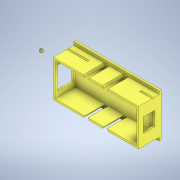
# Autodesk Inventor part: usbHubCaseForTripodClamp
Saved by Autodesk Inventor 2021.2 (Build 252289000, 289)
## iProperties
Created: 2021-02-17
Part Number: usbHubCaseForTripodClamp
Material: PC/ABS Plastic
Document SubType Name: Modeling
Designer: robst
Density: 0.357273 g/cm^3
Appearance: Smooth - Yellow
Author: robst
Autodesk Inventor part; units mm, degrees
ref_plane "YZ Plane" through (0, 0, 0) normal (1, 0, 0) x (0, 1, 0)
ref_plane "XZ Plane" through (0, 0, 0) normal (0, 1, 0) x (-1, 0, 0)
ref_plane "XY Plane" through (0, 0, 0) normal (0, 0, 1) x (1, 0, 0)
sketch "Sketch1" plane through (0, 0, 0) normal (0, 0, 1) x (1, 0, 0)
  line L0 (-57.15, -29.21) -> (57.15, -29.21)
  line L1 (57.15, -29.21) -> (57.15, 29.21)
  line L2 (57.15, 29.21) -> (-57.15, 29.21)
  line L3 (-57.15, 29.21) -> (-57.15, -29.21)
  line L4 (-57.15, -29.21) -> (57.15, 29.21) construction
  line L5 (57.15, -29.21) -> (-57.15, 29.21) construction
  point P0 (0, 0)
  dimension "d0" = 58.42
  dimension "d1" = 114.3
  constraints: 12 end point, 2 midpoint, 2 parallel, 1 horizontal, 1 perpendicular
  measures "d0" distance of L2.end L0.start
  measures "d1" distance of L1.end L2.end
extrude "Extrusion1" add sketch "Sketch1" against normal blind 2.54
sketch "Sketch2" plane through (0, 0, 0) normal (0, 0, 1) x (1, 0, 0)
  line L0 (-57.15, -29.21) -> (-57.15, 29.21) projected
  line L1 (57.15, 29.21) -> (57.15, -29.21) projected
  line L2 (-57.15, 24.765) -> (57.15, 24.765)
  line L3 (57.15, 24.765) -> (57.15, 22.225)
  line L4 (57.15, 22.225) -> (-57.15, 22.225)
  line L5 (-57.15, 22.225) -> (-57.15, 24.765)
  line L6 (-57.15, -24.765) -> (57.15, -24.765)
  line L7 (57.15, -24.765) -> (57.15, -22.225)
  line L8 (57.15, -22.225) -> (-57.15, -22.225)
  line L9 (-57.15, -22.225) -> (-57.15, -24.765)
  point P0 (0, 0)
  point P1 (-57.15, -22.225)
  point P2 (57.15, -24.765)
  dimension "d4" = 2.54
  dimension "d5" = 2.54
  dimension "d6" = 22.225
  dimension "d7" = 22.225
  constraints: 16 end point, 4 parallel, 4 point on line, 2 horizontal, 2 perpendicular
  measures "d4" distance between parallel lines of L4 L2
  measures "d5" distance between parallel lines of L6 L8
  measures "d6" distance from line of L4 point (0, 0)
  measures "d7" distance from line of L8 point (0, 0)
extrude "Extrusion2" add sketch "Sketch2" along normal blind 27.432 contours L0 L8 L1 L6 | L0 L2 L1 L4
sketch "Sketch3" plane through (0, 0, -2.54) normal (0, 0, -1) x (-1, 0, 0)
  line L0 (-12.7, -25.4) -> (12.7, -25.4) construction
  line L1 (12.7, -25.4) -> (12.7, 25.4) construction
  line L2 (12.7, 25.4) -> (-12.7, 25.4) construction
  line L3 (-12.7, 25.4) -> (-12.7, -25.4) construction
  line L4 (-12.7, -25.4) -> (12.7, 25.4) construction
  line L5 (12.7, -25.4) -> (-12.7, 25.4) construction
  point P0 (0, 0)
  dimension "d10" = 25.4
  dimension "d11" = 50.8
  constraints: 12 end point, 4 coincident, 2 midpoint, 2 parallel, 1 horizontal, 1 perpendicular
  measures "d10" distance of L1.end L2.end
  measures "d11" distance of L2.end L0.start
hole "Hole1" at (12.7, 25.4, -2.54) at (-12.7, 25.4, -2.54) at (-12.7, -25.4, -2.54) at (12.7, -25.4, -2.54) direction (0, 0, 1) diameter 3.81 end through all clearance for "Flat Head Machine Screw (82)" size "#6" standard "Ansi Unified Screw Threads"
sketch "Sketch4" plane through (0, 0, 0) normal (0, 0, 1) x (1, 0, 0)
  circle A0 centre (-12.7, 25.4) radius 1.905 projected
  circle A1 centre (-12.7, 25.4) radius 3.81
  circle A2 centre (12.7, 25.4) radius 1.905 projected
  circle A3 centre (12.7, 25.4) radius 3.81
  circle A4 centre (12.7, -25.4) radius 1.905 projected
  circle A5 centre (12.7, -25.4) radius 3.81
  arc A6 (-14.4961, -24.765) -> (-10.9039, -24.765) centre (-12.7, -25.4) ccw projected
  circle A7 centre (-12.7, -25.4) radius 3.81
  point P0 (0, 0)
  dimension "d19" = 7.62
  constraints: 4 centre point, 4 coincident, 3 equal radius
  measures "d19" diameter of A1
extrude "Extrusion3" cut sketch "Sketch4" along normal through all contours A0 | A1 | A2 | A3 | A4 | A5 | A7
sketch "Sketch5" plane through (57.15, -29.21, -2.54) normal (1, 0, 0) x (0, 0, -1)
  line L0 (-29.972, 53.975) -> (-29.972, 51.435) projected
  line L1 (-2.54, 51.435) -> (-2.54, 6.985) projected
  line L2 (-29.972, 51.435) -> (-2.54, 51.435)
  line L3 (-2.54, 51.435) -> (-2.54, 6.985)
  line L4 (-2.54, 6.985) -> (-29.972, 6.985)
  line L5 (-29.972, 6.985) -> (-29.972, 51.435)
  point P0 (-2.54, 29.21)
  constraints: 8 end point, 2 parallel, 1 horizontal, 1 perpendicular
extrude "Extrusion4" add sketch "Sketch5" against normal blind 2.54
sketch "Sketch6" plane through (57.15, -29.21, -2.54) normal (1, 0, 0) x (0, 0, -1)
  line L0 (-2.54, 51.435) -> (-29.972, 51.435) projected
  line L1 (-2.54, 6.985) -> (-2.54, 51.435) projected
  line L2 (-29.972, 6.985) -> (-2.54, 6.985) projected
  line L3 (-29.972, 51.435) -> (-29.972, 53.975) construction
  line L4 (-29.972, 51.435) -> (-2.54, 6.985) construction
  line L5 (-2.54, 51.435) -> (-29.972, 6.985) construction
  line L6 (-23.876, 19.685) -> (-8.636, 19.685)
  line L7 (-8.636, 19.685) -> (-8.636, 38.735)
  line L8 (-8.636, 38.735) -> (-23.876, 38.735)
  line L9 (-23.876, 38.735) -> (-23.876, 19.685)
  line L10 (-23.876, 19.685) -> (-8.636, 38.735) construction
  line L11 (-8.636, 19.685) -> (-23.876, 38.735) construction
  point P0 (-2.54, 29.21)
  point P1 (-16.256, 29.21)
  dimension "d24" = 15.24
  dimension "d25" = 19.05
  constraints: 16 end point, 3 midpoint, 2 parallel, 1 horizontal, 1 perpendicular
  measures "d24" distance of L7.end L8.end
  measures "d25" distance of L6.end L7.end
extrude "Extrusion5" cut sketch "Sketch6" against normal up to surface (2.54 mm away)
sketch "Sketch7" plane through (-57.15, -29.21, -2.54) normal (-1, 0, 0) x (0, 0, 1)
  line L0 (2.54, 51.435) -> (29.972, 51.435) projected
  line L1 (29.972, 6.985) -> (29.972, 51.435) projected
  line L2 (2.54, 6.985) -> (29.972, 6.985) projected
  line L3 (2.54, 51.435) -> (2.54, 6.985) projected
  line L4 (2.54, 6.985) -> (2.54, 51.435) construction
  line L5 (29.972, 6.985) -> (2.54, 6.985) construction
  line L6 (2.54, 51.435) -> (29.972, 6.985) construction
  line L7 (2.54, 51.435) -> (29.972, 51.435) construction
  line L8 (29.972, 51.435) -> (2.54, 6.985) construction
  line L9 (5.461, 13.97) -> (27.051, 13.97)
  line L10 (27.051, 13.97) -> (27.051, 44.45)
  line L11 (27.051, 44.45) -> (5.461, 44.45)
  line L12 (5.461, 44.45) -> (5.461, 13.97)
  line L13 (5.461, 13.97) -> (27.051, 44.45) construction
  line L14 (27.051, 13.97) -> (5.461, 44.45) construction
  point P0 (2.54, 29.21)
  point P1 (16.256, 29.21)
  dimension "d28" = 30.48
  dimension "d29" = 21.59
  constraints: 16 end point, 3 midpoint, 2 parallel, 2 perpendicular
  measures "d28" distance of L11.end L9.start
  measures "d29" distance of L10.end L11.end
extrude "Extrusion6" add sketch "Sketch7" against normal blind 2.54
sketch "Sketch8" plane through (57.15, -29.21, -2.54) normal (1, 0, 0) x (0, 0, -1)
  line L0 (-2.54, 53.975) -> (-29.972, 53.975) projected
  line L1 (-29.972, 53.975) -> (-2.54, 53.975) projected
  line L2 (-12.192, 53.975) -> (-10.922, 52.705)
  line L3 (-10.922, 52.705) -> (-9.652, 53.975)
  line L4 (-9.652, 53.975) -> (-12.192, 53.975)
  line L5 (-29.972, 4.445) -> (-29.972, 53.975) projected
  point P0 (-2.54, 29.21)
  dimension "d32" = 90
  dimension "d33" = 135
  dimension "d34" = 1.27
  dimension "d35" = 19.05
  constraints: 6 end point, 2 point on line, 1 collinear
  measures "d32" angle of L3 L2
  measures "d33" angle of L2 L0
  measures "d34" distance from line of L2.end L0
  measures "d35" distance from line of L2.end L5
extrude "Extrusion7" cut sketch "Sketch8" against normal blind 16.51
mirror "Mirror1" about plane through (0, 0, 0) normal (0, 1, 0) of "Extrusion7"
sketch "Sketch9" plane through (-57.15, -29.21, -2.54) normal (-1, 0, 0) x (0, 0, 1)
  line L0 (9.652, 53.975) -> (10.922, 52.705) projected
  line L1 (10.922, 52.705) -> (12.192, 53.975) projected
  line L2 (2.54, 53.975) -> (29.972, 53.975) projected
  line L3 (12.192, 53.975) -> (10.922, 52.705)
  line L4 (9.652, 53.975) -> (10.922, 52.705) projected
  line L5 (10.922, 52.705) -> (9.652, 53.975)
  line L6 (9.652, 53.975) -> (12.192, 53.975)
  line L7 (2.54, 53.975) -> (29.972, 53.975) projected
  point P0 (2.54, 29.21)
  constraints: 6 end point, 2 collinear
extrude "Extrusion8" cut sketch "Sketch9" against normal blind 27.94
mirror "Mirror2" about plane through (0, 0, 0) normal (0, 1, 0) of "Extrusion8"
equation "\"d0\" = usbHolderWidth"
equation "\"d1\" = usbHolderLength"
equation "\"d2\" = usbHolderWallThickness"
equation "\"d4\" = usbHolderWallThickness"
equation "\"d5\" = usbHolderWallThickness"
equation "\"d6\" = 0.5 * usbHubWidth"
equation "\"d7\" = 0.5 * usbHubWidth"
equation "\"d8\" = usbHubDepth"
equation "\"d10\" = holePatternLength"
equation "\"d11\" = holePatternWidth"
equation "\"d22\" = usbHolderWallThickness"
equation "\"d26\" = usbHolderWallThickness"
equation "\"d30\" = usbHolderWallThickness"
equation "\"usbHolderWallThickness\" = 2.54"
equation "\"usbHubWidth\" = 44.45"
equation "\"usbHubDepth\" = 27.432"
equation "\"usbHubLength\" = 109.22"
equation "\"usbHolderWidth\" = 58.42"
equation "\"usbHolderLength\" = usbHubLength + 2 * usbHolderWallThickness"
equation "\"holePatternLength\" = 25.4"
equation "\"holePatternWidth\" = 50.8"
body "Solid1"
